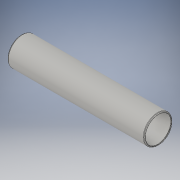
# Autodesk Inventor part: 09R-5.31250SR
Saved by Autodesk Inventor 2016 SP1 (Build 200210100, 210)
## iProperties
Category: PARTsolutions
Company: BIMBA
Created: 2017-03-15
Part Number: 09R-5.31250SR
Material: Generic
Catalog Web Link: www.cadenas.de
Description: Tube-Original Line - Standard Air Cylinders
Vendor: BIMBA
Document SubType Name: Standard Catalog Part
Designer: 589013
Manufacturer: BIMBA
Mass: 6.31713 g
Surface Area: 238.885 cm^2
Volume: 6.31713 cm^3
Density: 1 g/cm^3
Appearance: PSOLRGB-180-180-180
PSOL_IDENT_0: {$CADENAS_DATA\23d-libs\bimba\bimba\bimba_imperial\bimba_full_line\original_line_cylinders\standard_
PSOL_IDENT_1: air_cylinders\tube.prj},194 {VTYP=3D},{NB=09R-5.31250SR},{LINA=09R-5.31250SR},{NN=Tube},{DATE=09.11.
PSOL_IDENT_2: 2016 07:55:11},{GEOMDATE=18.02.2011 00:00:00},{VERSION=},{LINEID=60},{LINESUBID=-1},{WBVAR=MNT,ACTIN
PSOL_IDENT_3: G,NR,L,FOURHOLES,SR}  {NB=09R-5.31250SR},{LINA=09R-5.31250SR},{KT=DUMMY},{PN=09R-5.31250SR},{BORE=1.
PSOL_IDENT_4: 06250000},{BOREPN=09},{MNT=},{MNTALG='' , 'Front Nose' , 'BF' , 'Front Block' , 'BFT' , 'Front Trunn
PSOL_IDENT_5: ion' , 'A' , 'Adjustable Stroke'},{ACTING=R},{ACTINGALG= '' , 'Single Acting' , 'R' , 'Reverse/Doubl
PSOL_IDENT_6: e Acting' },{NR=},{NRALG= '' , 'N/A' },{L=5.3125},{OD=1.1130},{ODN=1.1130},{ODP=1.1130},{ODB=1.1410}
PSOL_IDENT_7: ,{ID=1.0715},{DV=0.00000000},{LV=0.00000000},{LV1=0.00000000},{G=0.0300},{FOURHOLES=0},{AA=0.3750},{
PSOL_IDENT_8: BB=0.0940},{SR=SR},{SRALG= 'C' , 'Carbon Steel Rod' , 'SR' , '303 Stainless Steel Rod' , '' , '303 S
PSOL_IDENT_9: tainless Steel Rod'}
NN: Tube
NT: Original Line - Standard Air Cylinders
NB: 09R-5.31250SR
NBSYN: $PN.
LINA: 09R-5.31250SR
BORE: 1 1/16
BOREPN: 09
MNT: Front Nose
MNTALG: '' , 'Front Nose' , 'BF' , 'Front Block' , 'BFT' , 'Front Trunnion' , 'A' , 'Adjustable Stroke'
ACTING: Reverse/Double Acting
NR: N/A
L: 5.3125
ODN: 1.1130
ODP: 1.1130
ODB: 1.1410
ID: 1.0715
DV: 0.00000000
LV: 0.00000000
LV1: 0.00000000
G: 0.0300
FOURHOLES: 0
AA: 0.3750
BB: 0.0940
SR: 303 Stainless Steel Rod
SUPPLIER: BIMBA
ARTICLENO: 09R-5.31250SR
BOMINFO: 09R-5.31250SR
CREATOR: CADENAS GmbH
Title: 09R-5.31250SR
Author: Cadenas PARTsolutions
Comments: Original Line - Standard Air Cylinders
Autodesk Inventor part; units mm, degrees
sketch "Sketch_1" plane through (0, 0, 0) normal (0, 0, 1) x (1, 0, 0)
  line L0 (134.9375, 0) -> (0, 0)
  arc A0 (-0.6395, 13.2842) -> (-0.6395, 13.1046) centre (-0.5497, 13.1944) ccw
  line L1 (-0.6395, 13.1046) -> (-0.381, 12.846)
  line L2 (-0.381, 12.846) -> (0, 12.846)
  line L3 (0, 12.846) -> (0.762, 13.6081)
  line L4 (0.762, 13.6081) -> (134.1755, 13.6081)
  line L5 (134.1755, 13.6081) -> (134.9375, 12.846)
  line L6 (134.9375, 12.846) -> (135.3185, 12.846)
  line L7 (135.3185, 12.846) -> (135.577, 13.1046)
  arc A1 (135.577, 13.1046) -> (135.577, 13.2842) centre (135.4872, 13.1944) ccw
  line L8 (135.577, 13.2842) -> (134.9493, 13.9119)
  arc A2 (134.9493, 13.9119) -> (134.4104, 14.1351) centre (134.4105, 13.3731) ccw
  line L9 (134.4104, 14.1351) -> (0.527, 14.1351)
  arc A3 (0.527, 14.1351) -> (-0.0118, 13.9119) centre (0.527, 13.3731) ccw
  line L10 (-0.0118, 13.9119) -> (-0.6395, 13.2842)
  constraints: 22 end point, 8 point on circle, 4 centre point
revolve "Revolution1" add sketch "Sketch_1" angle 360 about axis through (134.9375, 0, 0) along (1, 0, 0)
ref_plane "cp1_XY" through (67.4688, 14.1351, 0) normal (1, 0, 0) x (0, 0, -1)
ref_plane "cp1_YZ" through (67.4688, 14.1351, 0) normal (0, 0, -1) x (0, 1, 0)
ref_plane "cp1_ZX" through (67.4688, 14.1351, 0) normal (0, 1, 0) x (1, 0, 0)
ref_plane "cp2_XY" through (67.4688, 0, -14.1351) normal (1, 0, 0) x (0, 0, -1)
ref_plane "cp2_YZ" through (67.4688, 0, -14.1351) normal (0, 0, -1) x (0, 1, 0)
ref_plane "cp2_ZX" through (67.4688, 0, -14.1351) normal (0, 1, 0) x (1, 0, 0)
ref_plane "cp3_XY" through (67.4688, -14.1351, 0) normal (1, 0, 0) x (0, 0, -1)
ref_plane "cp3_YZ" through (67.4688, -14.1351, 0) normal (0, 0, -1) x (0, 1, 0)
ref_plane "cp3_ZX" through (67.4688, -14.1351, 0) normal (0, 1, 0) x (1, 0, 0)
ref_plane "cp4_XY" through (67.4688, 0, 14.1351) normal (1, 0, 0) x (0, 0, -1)
ref_plane "cp4_YZ" through (67.4688, 0, 14.1351) normal (0, 0, -1) x (0, 1, 0)
ref_plane "cp4_ZX" through (67.4688, 0, 14.1351) normal (0, 1, 0) x (1, 0, 0)
ref_plane "tube_front_XY" through (0, 0, 0) normal (1, 0, 0) x (0, 0, -1)
ref_plane "tube_front_YZ" through (0, 0, 0) normal (0, 0, -1) x (0, 1, 0)
ref_plane "tube_front_ZX" through (0, 0, 0) normal (0, 1, 0) x (1, 0, 0)
ref_plane "tube_rear_XY" through (134.9375, 0, 0) normal (1, 0, 0) x (0, 0, -1)
ref_plane "tube_rear_YZ" through (134.9375, 0, 0) normal (0, 0, -1) x (0, 1, 0)
ref_plane "tube_rear_ZX" through (134.9375, 0, 0) normal (0, 1, 0) x (1, 0, 0)
body "Solid1"
